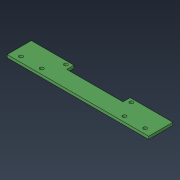
# Autodesk Inventor part: Eyeboard
Saved by Autodesk Inventor 2022.1 (Build 261234020, 234B)
## iProperties
Part Number: Eyeboard
Material: Phenolharz
Document SubType Name: Modeling
Designer: rYan
Mass: 2.18658 g
Surface Area: 23.6457 cm^2
Volume: 1.58448 cm^3
Density: 1.38 g/cm^3
Appearance: Glatt - waldgrün
Author: rYan
Autodesk Inventor part; units mm, degrees
ref_plane "YZ Plane" through (0, 0, 0) normal (1, 0, 0) x (0, 1, 0)
ref_plane "XZ Plane" through (0, 0, 0) normal (0, 1, 0) x (-1, 0, 0)
ref_plane "XY Plane" through (0, 0, 0) normal (0, 0, 1) x (1, 0, 0)
sketch "Skizze1" plane through (0, 0, 0) normal (0, 0, 1) x (1, 0, 0)
  line L0 (-41, -7) -> (41, -7)
  line L1 (41, -7) -> (41, 7)
  line L2 (-41, 7) -> (-41, -7)
  line L3 (-41, -7) -> (41, 7) construction
  line L4 (41, -7) -> (-41, 7) construction
  line L5 (16.3, 7) -> (16.3, 2.8)
  line L6 (16.3, 2.8) -> (-16.3, 2.8)
  line L7 (-16.3, 2.8) -> (-16.3, 7)
  line L8 (41, 7) -> (16.3, 7)
  line L9 (-16.3, 7) -> (-41, 7)
  line L10 (0, 9.8) -> (0, -9.8) projected
  point P0 (0, 0)
  dimension "d0" = 82
  dimension "d1" = 14
  dimension "d13" = 4.2
  dimension "d14" = 32.6
  constraints: 20 end point, 4 parallel, 2 midpoint, 1 horizontal, 1 perpendicular, 2 other
  measures "d0" distance of L2.start L1.end
  measures "d1" distance of L1.end L0.end
  measures "d13" distance between parallel lines of L9 L6
  measures "d14" distance of L5.end L6.end
extrude "Extrusion1" add sketch "Skizze1" along normal blind 1.6
sketch "Skizze2" plane through (0, 0, 1.6) normal (0, 0, 1) x (1, 0, 0)
  line L0 (0, 9.8) -> (0, -9.8) projected
  line L1 (-57.4, 0) -> (57.4, 0) projected
  line L2 (-19, 5) -> (19, 5) construction
  line L3 (-16.3, 7) -> (-41, 7) projected
  point P0 (0, 0)
  dimension "d4" = 38
  dimension "d15" = 2
  constraints: 2 coincident, 2 end point, 1 horizontal, 1 symmetric about line
  measures "d4" distance of L2.start L2.end
  measures "d15" distance between parallel lines of L2 L3
hole "Bohrung1" at (-19, 5, 1.6) at (19, 5, 1.6) direction (0, 0, -1) diameter 2.1 end through all
sketch "Skizze3" plane through (0, 0, 1.6) normal (0, 0, 1) x (1, 0, 0)
  line L0 (-41, -7) -> (41, -7) projected
  line L1 (0, 9.8) -> (0, -9.8) projected
  line L2 (-36, -4) -> (-24, -4) construction
  line L3 (24, -4) -> (36, -4) construction
  point P0 (0, 0)
  dimension "d16" = 3
  dimension "d17" = 24
  dimension "d18" = 12
  constraints: 4 end point, 2 horizontal, 2 symmetric about line, 1 collinear
  measures "d16" distance between parallel lines of L2 L0
  measures "d17" distance from line of L2.end L1
  measures "d18" distance of L2.start L2.end
hole "Bohrung2" at (-36, -4, 1.6) at (-24, -4, 1.6) at (24, -4, 1.6) at (36, -4, 1.6) direction (0, 0, -1) diameter 2.1 end through all
